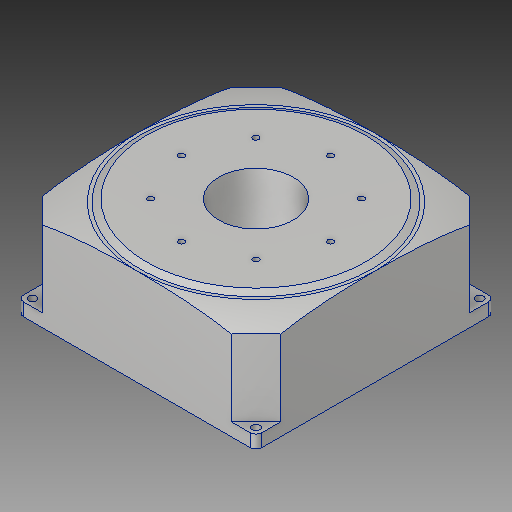
# Autodesk Inventor part: DT240
Saved by Autodesk Inventor 2019 (Build 230136000, 136)
## iProperties
Created: 2016-09-25
Part Number: DT240
Material: Aluminum 6061
Document SubType Name: Modeling
Designer: Eivind
Density: 2.7 g/cm^3
Appearance: Aluminum - Flat
Mass: 13851.6 g
Surface Area: 2183.73 cm^2
Volume: 5130.23 cm^3
Author: Eivind
Autodesk Inventor part; units mm, degrees
ref_plane "YZ Plane" through (0, 0, 0) normal (1, 0, 0) x (0, 1, 0)
ref_plane "XZ Plane" through (0, 0, 0) normal (0, 1, 0) x (-1, 0, 0)
sketch "Sketch1" plane through (0, 0, 0) normal (0, 1, 0) x (-1, 0, 0)
  point P0 (0, 0)
sketch "Sketch2" plane through (0, 0, 0) normal (0, 1, 0) x (-1, 0, 0)
  line L0 (120, 120) -> (-120, 120)
  line L1 (-120, 120) -> (-120, -120)
  line L2 (-120, -120) -> (120, -120)
  line L3 (120, -120) -> (120, 120)
  circle A0 centre (0, 0) radius 37.5
  dimension "d0" = 240
  dimension "d1" = 240
  dimension "d3" = 120
  dimension "d4" = 120
  dimension "d5" = 75
  constraints: 8 end point, 2 parallel, 1 centre point, 1 coincident, 1 horizontal, 1 perpendicular
  measures "d0" distance of L1.end L2.end
  measures "d1" distance of L0.end L1.end
  measures "d3" distance from line of L3 point (0, 0)
  measures "d4" distance from line of L0 point (0, 0)
  measures "d5" diameter of A0
extrude "Extrusion1" add sketch "Sketch2" along normal blind 100
fillet "Fillet1" radius 6 1 edges at (-120, 50, -120)
fillet "Fillet2" radius 6 1 edges at (120, 50, -120)
fillet "Fillet3" radius 6 1 edges at (120, 50, 120)
fillet "Fillet4" radius 6 1 edges at (-120, 50, 120)
sketch "Sketch3" plane through (0, 100, 0) normal (0, 1, 0) x (1, 0, 0)
  line L0 (0, 0) -> (75, 0) construction
  point P0 (-75, 0)
  point P1 (0, 75)
  point P2 (0, 75)
  point P3 (0, -75)
  point P4 (-53.033, 53.033)
  point P5 (-53.033, 53.033)
  point P6 (53.033, 53.033)
  point P7 (53.033, -53.033)
  point P8 (-53.033, -53.033)
  dimension "d14" = 53.033
  dimension "d15" = 53.033
  dimension "d16" = 53.033
  dimension "d17" = 53.033
  dimension "d18" = 53.033
  dimension "d19" = 53.033
  constraints: 2 coincident, 2 end point, 1 horizontal
  measures "d14" horizontal distance of L0.start point (-53.033, 53.033)
  measures "d15" horizontal distance of L0.start point (-53.033, 53.033)
  measures "d16" horizontal distance of point (53.033, 53.033) L0.start
  measures "d17" horizontal distance of point (53.033, 53.033) L0.start
  measures "d18" horizontal distance of L0.start point (53.033, -53.033)
  measures "d19" horizontal distance of point (53.033, -53.033) L0.start
hole "Hole1" at (-75, 100, 0) at (75, 100, 0) at (0, 100, -75) at (0, 100, 75) at (-53.033, 100, -53.033) at (53.033, 100, -53.033) at (53.033, 100, 53.033) at (-53.033, 100, 53.033) direction (0, -1, 0) diameter 6 depth 10 tip angle 118
sketch "Sketch4" plane through (0, 100, 0) normal (0, 1, 0) x (1, 0, 0)
  point P0 (0, 0)
  point P1 (-112.5, 112.5)
  point P2 (-112.5, -112.5)
  point P3 (112.5, -112.5)
  point P4 (112.5, 112.5)
  dimension "d34" = 112.5
  dimension "d35" = 112.5
  measures "d34" horizontal distance of point (0, 0) point (112.5, -112.5)
  measures "d35" horizontal distance of point (112.5, -112.5) point (0, 0)
hole "Hole2" at (-112.5, 100, -112.5) at (-112.5, 100, 112.5) at (112.5, 100, 112.5) at (112.5, 100, -112.5) direction (0, -1, 0) diameter 8 end through all
sketch "Sketch5" plane through (0, 100, 0) normal (0, 1, 0) x (1, 0, 0)
  line L0 (95, 120) -> (120, 95)
  line L1 (120, -114) -> (120, 114) projected
  line L2 (95, 120) -> (130.3553, 120) construction
  line L3 (114, 120) -> (-114, 120) projected
  line L4 (-95, 120) -> (-120, 95)
  line L5 (-120, 114) -> (-120, -114) projected
  line L6 (-95, 120) -> (-59.6447, 120) construction
  line L7 (95, 120) -> (120, 120)
  line L8 (120, 120) -> (120, 95)
  line L9 (-95, 120) -> (-120, 120)
  line L10 (-120, 120) -> (-120, 95)
  point P0 (0, 0)
  dimension "d36" = 45
  dimension "d38" = 135
  constraints: 16 end point, 5 point on line, 2 equal length, 2 horizontal, 2 perpendicular
  measures "d36" angle of L0 L2
  measures "d38" angle of L4 L6
extrude "Extrusion2" cut sketch "Sketch5" against normal blind 87 contours L3 L7 L8 L1 L0
sketch "Sketch6" plane through (0, 100, 0) normal (0, 1, 0) x (1, 0, 0)
  line L0 (114, 120) -> (-114, 120)
  line L1 (-95, 120) -> (-120, 95)
  line L2 (-120, 114) -> (-120, -114)
  line L3 (-95, 120) -> (-59.6447, 120) construction
  line L4 (-95, 120) -> (-120, 120)
  line L5 (-120, 120) -> (-120, 95)
  point P0 (0, 0)
  dimension "d41" = 135
  constraints: 12 end point, 2 point on line, 1 equal length, 1 horizontal, 1 perpendicular
  measures "d41" angle of L1 L3
extrude "Extrusion3" cut sketch "Sketch6" against normal blind 87
sketch "Sketch7" plane through (0, 100, 0) normal (0, 1, 0) x (1, 0, 0)
  line L0 (120, -114) -> (120, 95) projected
  line L1 (120, -95) -> (95, -120)
  line L2 (-114, -120) -> (114, -120) projected
  line L3 (120, -95) -> (155.3553, -95) construction
  line L4 (120, -95) -> (120, -120)
  line L5 (120, -120) -> (95, -120)
  point P0 (0, 0)
  dimension "d44" = 135
  constraints: 8 end point, 2 point on line, 1 collinear, 1 equal length, 1 horizontal, 1 vertical
  measures "d44" angle of L1 L3
extrude "Extrusion4" cut sketch "Sketch7" against normal blind 87
sketch "Sketch8" plane through (0, 100, 0) normal (0, 1, 0) x (1, 0, 0)
  line L0 (-120, 95) -> (-120, -114) projected
  line L1 (-120, -95) -> (-95, -120)
  line L2 (-114, -120) -> (95, -120) projected
  line L3 (-120, -95) -> (-84.6447, -95) construction
  line L4 (-95, -120) -> (-120, -120)
  line L5 (-120, -120) -> (-120, -95)
  point P0 (0, 0)
  dimension "d47" = 45
  constraints: 8 end point, 2 perpendicular, 2 point on line, 1 equal length, 1 horizontal
  measures "d47" angle of L1 L3
extrude "Extrusion5" cut sketch "Sketch8" against normal blind 87
sketch "Sketch9" plane through (0, 100, 0) normal (0, 1, 0) x (1, 0, 0)
  circle A0 centre (0, 0) radius 116.75
  line L0 (120, 120) -> (-120, 120)
  line L1 (-120, 120) -> (-120, -120)
  line L2 (-120, -120) -> (120, -120)
  line L3 (120, -120) -> (120, 120)
  dimension "d50" = 233.5
  dimension "d53" = 240
  dimension "d54" = 240
  constraints: 8 end point, 2 parallel, 1 centre point, 1 coincident, 1 horizontal, 1 perpendicular
  measures "d50" diameter of A0
  measures "d53" distance of L2.end L1.end
  measures "d54" distance of L1.end L0.end
extrude "Extrusion6" cut sketch "Sketch9" against normal blind 3
ref_plane "Work Plane1" through (0, 0, 0) normal (0.7071, 0, -0.7071) x (0, 1, 0)
sketch "Sketch10" plane through (0, 0, 0) normal (0.7071, 0, -0.7071) x (0, 1, 0)
  line L0 (97, 116.75) -> (135.5145, 116.75) construction
  line L1 (97, -116.75) -> (97, 116.75) projected
  line L2 (97, 116.75) -> (151.2428, 116.75) construction
  line L3 (-153.1261, 0) -> (197.3136, 0) projected
  arc A0 (97, 120) -> (84.2851, 167.4528) centre (-101.0801, 92.3545) ccw
  line L4 (97, 120) -> (84.2851, 167.4528) construction
  line L5 (97, 120) -> (146.1267, 120) construction
  line L6 (84.2851, 167.4528) -> (97, 167.4528)
  line L7 (97, 167.4528) -> (97, 120)
  line L8 (97, 17.6777) -> (97, 152.028) projected
  line L9 (100, -116.75) -> (100, 116.75) projected
  point P0 (0, 0)
  dimension "d62" = 105
  dimension "d63" = 200
  dimension "d64" = 120
  dimension "d65" = 3
  constraints: 12 end point, 4 horizontal, 2 point on circle, 1 centre point, 1 collinear, 1 equal length
  measures "d62" angle of L5 L4
  measures "d63" radius of A0
  measures "d64" distance from line of L3 L4.start
  measures "d65" distance between parallel lines of L9 L7
revolve "Revolution1" cut sketch "Sketch10" angle 360 about axis through (0, -10, 0) along (0, 1, 0)
sketch "Sketch11" plane through (0, 0, 0) normal (0.7071, 0, -0.7071) x (0, 1, 0)
  line L0 (97, -116.75) -> (97, 116.75) projected
  line L1 (97, 116.75) -> (100, 110.3165)
  line L2 (100, -116.75) -> (100, 116.75) projected
  line L3 (97, 116.75) -> (104.0986, 116.75) construction
  line L4 (100, 110.3165) -> (100, 116.75)
  line L5 (100, 116.75) -> (97, 116.75)
  line L6 (-21.7182, 0) -> (130.3093, 0) projected
  point P0 (0, 0)
  dimension "d66" = 65
  constraints: 8 end point, 1 collinear, 1 equal length, 1 horizontal, 1 perpendicular, 1 point on line
  measures "d66" angle of L1 L3
revolve "Revolution2" cut sketch "Sketch11" angle 360 about axis through (0, -10, 0) along (0, 1, 0) contours L5 L2 L1
body "Solid1"
